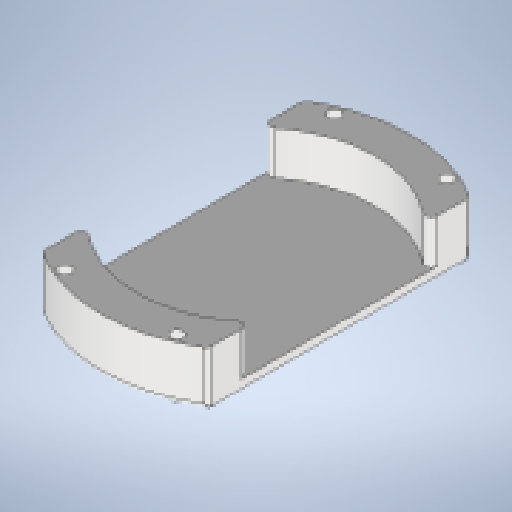
# Autodesk Inventor part: base_part8
Saved by Autodesk Inventor 2024 (Build 280153000, 153)
## iProperties
Created: 2025-02-22
Part Number: base_part8
Material: 一般
Document SubType Name: Modeling
Designer: tanoue_kota
Density: 1 g/cm^3
Appearance: 既定
Author: tanoue_kota
Autodesk Inventor part; units mm, degrees
ref_plane "YZ Plane" through (0, 0, 0) normal (1, 0, 0) x (0, 1, 0)
ref_plane "XZ Plane" through (0, 0, 0) normal (0, 1, 0) x (-1, 0, 0)
ref_plane "XY Plane" through (0, 0, 0) normal (0, 0, 1) x (1, 0, 0)
sketch "スケッチ1" plane through (0, 0, 0) normal (0, 1, 0) x (-1, 0, 0)
  circle A0 centre (0, 0) radius 52
  line L0 (27.9396, 43.8564) -> (27.9396, -43.8564)
  line L1 (27.9396, -43.8564) -> (0, 0)
  line L2 (0, 0) -> (52, 0)
  line L3 (27.9396, 43.8564) -> (0, 0)
  line L4 (0, 52) -> (0, -52)
  line L5 (-27.9396, 43.8564) -> (-27.9396, -43.8564)
  line L6 (-27.9396, -43.8564) -> (0, 0)
  line L7 (-27.9396, 43.8564) -> (0, 0)
  dimension "d0" = 104
  dimension "d1" = 57.5
  constraints: 16 end point, 5 point on circle, 2 symmetric about line, 2 vertical, 1 centre point, 1 coincident, 1 perpendicular
  measures "d0" diameter of A0
  measures "d1" angle of L2 L1
extrude "押し出し1" add sketch "スケッチ1" along normal blind 18.35 contours L3 L4 A0 | L0 L2 L3 | L1 L2 L0 | A0 L4 L1 | L4 L7 A0 | L4 A0 L6 | L6 L5 L7
sketch "スケッチ2" plane through (0, 18.35, 0) normal (0, 1, 0) x (1, 0, 0)
  circle A0 centre (0, 0) radius 39.9
  dimension "d4" = 79.8
  constraints: 1 centre point, 1 coincident
  measures "d4" diameter of A0
extrude "押し出し2" cut sketch "スケッチ2" against normal blind 14.6
sketch "スケッチ3" plane through (0, 0, 0) normal (0, -1, 0) x (1, 0, 0)
  line L0 (0, 0) -> (0, 52)
  arc A0 (27.9396, 43.8564) -> (-27.9396, 43.8564) centre (0, 0) ccw projected
  line L1 (0, 0) -> (19.8995, 48.0417)
  line L2 (0, 0) -> (27.9396, 0)
  line L3 (27.9396, -28.4849) -> (27.9396, 28.4849) projected
  point P0 (18.7515, 45.2701)
  point P1 (-18.7515, 45.2701)
  point P2 (18.7515, -45.2701)
  point P3 (-18.7515, -45.2701)
  dimension "d8" = 98
  dimension "d7" = 22.5
  constraints: 6 end point, 3 symmetric about line, 2 point on circle, 1 coincident, 1 midpoint, 1 point on line, 1 vertical, 3 other
  measures "d7" angle of L0 L1
hole "穴1" at (18.7515, 0, 45.2701) at (-18.7515, 0, 45.2701) at (-18.7515, 0, -45.2701) at (18.7515, 0, -45.2701) direction (0, 1, 0) diameter 4.2 end through all
fillet "フィレット1" radius 1 16 edges at (0, 18.35, 39.9) (0, 18.35, -39.9) (0, 18.35, 52) (27.9396, 3.75, 0) (27.9396, 0, 0) (27.9396, 11.05, 28.4849) (27.9396, 11.05, -28.4849) (27.9396, 9.175, 43.8564) (-27.9396, 9.175, 43.8564) (-27.9396, 11.05, 28.4849) (-27.9396, 11.05, -28.4849) (27.9396, 9.175, -43.8564) (0, 18.35, -52) (-27.9396, 9.175, -43.8564) (-27.9396, 3.75, 0) (-27.9396, 0, 0)
